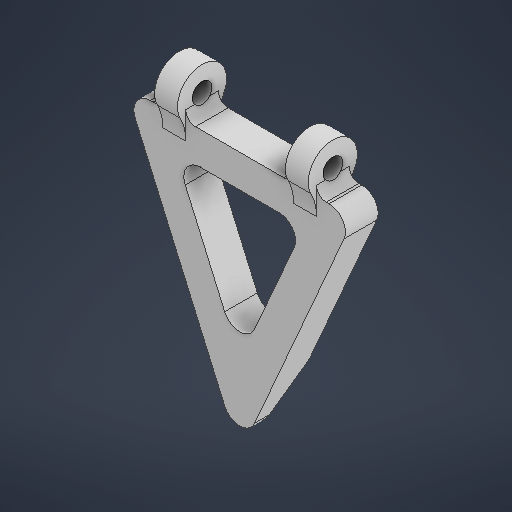
# Autodesk Inventor part: trojúhleník_FF
Saved by Autodesk Inventor 2026 (Build 300175050, 175E)
## iProperties
Created: 2026-02-24
Part Number: trojúhleník_FF
Material: Všeobecné
Document SubType Name: Modeling
Designer: marti
Density: 1 g/cm^3
Appearance: Výchozí
Author: marti
Autodesk Inventor part; units mm, degrees
ref_plane "XZ Plane" through (0, 0, 0) normal (0, 1, 0) x (-1, 0, 0)
sketch "Náčrt1" plane through (0, 0, 0) normal (0, 0, 1) x (1, 0, 0)
  line L0 (-35, 35) -> (35, 35)
  line L1 (-35, 35) -> (0, -45)
  line L2 (0, -45) -> (35, 35)
  line L3 (0, 51) -> (0, -61) projected
  line L4 (-49, 0) -> (49, 0) projected
  line L5 (19.7098, 25) -> (-19.7098, 25)
  line L6 (-19.7098, 25) -> (0, -20.0511)
  line L7 (0, -20.0511) -> (19.7098, 25)
  point P0 (0, 0)
  dimension "d3" = 70
  dimension "d36" = 80
  dimension "d37" = 35
  dimension "d38" = 10
  constraints: 12 end point, 1 parallel, 1 point on line, 1 symmetric about line, 2 other
  measures "d3" distance of L0.start L0.end
  measures "d36" distance from line of L0 L1.end
  measures "d37" distance between parallel lines of L0 L4
  measures "d38" distance between parallel lines of L2 L7
extrude "Vysunutí1" add sketch "Náčrt1" along normal mid plane 10 contours L0 L3 L5 L6 L4 L1 | L0 L2 L4 L7 L5 L3 | L4 L6 L3 L1 | L3 L7 L4 L2
fillet "Zaoblení1" radius 5 6 edges at (-35, 35, 0) (35, 35, 0) (0, -45, 0) (0, -20.0511, 0) (-19.7098, 25, 0) (19.7098, 25, 0)
ref_plane "Pracovní rovina1" through (20, 0, 0) normal (1, 0, 0) x (0, 1, 0)
ref_plane "Pracovní rovina2" through (-20, 0, 0) normal (1, 0, 0) x (0, 1, 0)
sketch "Náčrt3" plane through (20, 0, 0) normal (1, 0, 0) x (0, 1, 0)
  line L0 (45, -5) -> (30, -5)
  line L1 (30, -5) -> (30, 5)
  line L2 (30, 5) -> (45, 5)
  line L3 (45, 5) -> (45, -5)
  line L4 (35, 5) -> (35, -5) projected
  point P0 (0, 0)
  dimension "d18" = 15
  dimension "d19" = 10
  dimension "d20" = 10
  constraints: 8 end point, 2 parallel, 1 horizontal, 1 perpendicular
  measures "d18" distance of L1.end L2.end
  measures "d19" distance of L0.end L1.end
  measures "d20" distance between parallel lines of L4 L3
sketch "Náčrt4" plane through (-20, 0, 0) normal (1, 0, 0) x (0, 1, 0)
  line L0 (35, -5) -> (27.9959, -5) projected
  line L1 (27.9959, -5) -> (27.9959, 5) projected
  line L2 (27.9959, 5) -> (35, 5) projected
  line L3 (35, 5) -> (35, -5) projected
  circle A0 centre (40, 0) radius 7.5
  point P0 (0, 0)
  point P1 (34.4098, -5)
  point P2 (34.4098, 5)
  dimension "d61" = 15
  constraints: 1 centre point
  measures "d61" diameter of A0
extrude "Vysunutí2" add sketch "Náčrt4" along normal mid plane 7
fillet "Zaoblení2" radius 3 2 edges at (-16.5, 35, 0) (-23.5, 35, 0)
ref_plane "Pracovní rovina7" through (23.5, 0, 0) normal (1, 0, 0) x (0, 0, -1)
sketch "Náčrt8" plane through (0, 0, 0) normal (1, 0, 0) x (0, 1, 0)
  line L0 (-54.0306, 0) -> (61.5051, 0) projected
  line L1 (0, 7) -> (0, -7) projected
  line L2 (27.9959, 5) -> (-34.5296, 5) projected
  arc A0 (38, -2.2361) -> (38, 2.2361) centre (40, 0) ccw projected
  line L3 (40, 0) -> (31.4495, 23.4923)
  line L4 (31.4495, 23.4923) -> (-33.0951, 0)
  line L5 (-33.0951, 0) -> (40, 0)
  line L6 (0, -7) -> (0, 7)
  line L7 (27.9959, -5) -> (-34.5296, -5)
  arc A1 (38, -2.2361) -> (38, 2.2361) centre (40, 0) ccw
  line L8 (40, 0) -> (31.4495, -23.4923)
  line L9 (31.4495, -23.4923) -> (-33.0951, 0)
  point P0 (0, 0)
  point P1 (-19.3577, 5)
  point P2 (0, 5)
  point P3 (0, -5)
  point P4 (-19.3577, -5)
  dimension "d47" = 25
  dimension "d48" = 20
  dimension "d49" = 90
  dimension "d50" = 0
  constraints: 14 end point, 7 symmetric about line, 2 point on circle, 1 centre point, 1 perpendicular, 1 other
  measures "d47" distance of L3.start L3.end
  measures "d48" angle of L4 L5
  measures "d49" angle of L4 L3
  measures "d50" distance between parallel lines of L0 L5
ref_plane "Pracovní rovina6" through (10, 31.4495, -23.4923) normal (0, -0.342, -0.9397) x (-1, 0, 0)
sketch "Náčrt10" plane through (10, 31.4495, -23.4923) normal (0, -0.342, -0.9397) x (-1, 0, 0)
  line L0 (-47.61, -16.3764) -> (81.0156, -16.3764)
  line L1 (81.0156, -16.3764) -> (81.0156, -106.6518)
  line L2 (81.0156, -106.6518) -> (-47.61, -106.6518)
  line L3 (-47.61, -106.6518) -> (-47.61, -16.3764)
  point P0 (10, -37.5877)
  constraints: 8 end point, 2 parallel, 1 horizontal, 1 perpendicular
extrude "Vysunutí8" cut sketch "Náčrt10" along normal blind 10
fillet "Zaoblení3" radius 15 2 edges at (-20, 34.4098, -5) (-20, 34.4098, 5)
mirror "Zrcadlit1" about plane through (0, 0, 0) normal (1, 0, 0) of "Vysunutí2", "Zaoblení2", "Zaoblení3"
sketch "Náčrt5" plane through (23.5, 0, 0) normal (1, 0, 0) x (0, 0, -1)
  line L0 (5, 35) -> (5, 45) projected
  line L1 (5, 45) -> (-5, 45) projected
  line L2 (-5, 45) -> (-5, 35) projected
  line L3 (5, 35) -> (-5, 35) projected
  point P0 (0, 0)
  point P1 (0, 40)
hole "Díra1" at (23.5, 40, 0) direction (1, 0, 0) diameter 6 end through all both
